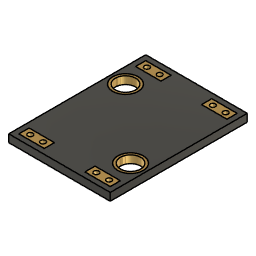
DC-DC Stepdown (Unfinished) v3 (Autodesk Fusion 360 design; units mm, degrees)
Autodesk Fusion 360 part; units mm, degrees
note: some values were not read from the file. Chosen so that the rebuilt part matches the saved one: which bodies a step acts on.
sketch "Sketch1" plane through (0, 0, 0) normal (0, 0, 1) x (1, 0, 0)
  line L0 (10, 13.5) -> (-10, 13.5)
  line L1 (-10, 13.5) -> (-10, -13.5)
  line L2 (-10, -13.5) -> (10, -13.5)
  line L3 (10, -13.5) -> (10, 13.5)
  line L4 (10, 13.5) -> (-10, -13.5) construction
  line L5 (-10, 13.5) -> (10, -13.5) construction
  line L6 (-9, -10.5) -> (-4, -10.5)
  line L7 (-4, -10.5) -> (-4, -12.5)
  line L8 (-4, -12.5) -> (-9, -12.5)
  line L9 (-9, -12.5) -> (-9, -10.5)
  line L10 (0, 13.5) -> (0, -13.5)
  line L11 (-10, 0) -> (10, 0)
  line L12 (9, -12.5) -> (4, -12.5)
  line L13 (4, -12.5) -> (4, -10.5)
  line L14 (9, -10.5) -> (9, -12.5)
  line L15 (4, -10.5) -> (9, -10.5)
  line L16 (-4, 12.5) -> (-9, 12.5)
  line L17 (-9, 12.5) -> (-9, 10.5)
  line L18 (-4, 10.5) -> (-4, 12.5)
  line L19 (-9, 10.5) -> (-4, 10.5)
  line L20 (9, 10.5) -> (4, 10.5)
  line L21 (4, 10.5) -> (4, 12.5)
  line L22 (9, 12.5) -> (9, 10.5)
  line L23 (4, 12.5) -> (9, 12.5)
  circle A0 centre (-7.75, -11.5) radius 0.5
  circle A1 centre (-5.25, -11.5) radius 0.5
  line L24 (-6.5, -10.5) -> (-6.5, -12.5)
  line L25 (6.5, -12.5) -> (6.5, -10.5)
  line L26 (6.5, 10.5) -> (6.5, 12.5)
  line L27 (-6.5, 10.5) -> (-6.5, 12.5)
  circle A2 centre (-7.75, 11.5) radius 0.5
  circle A3 centre (5.25, 11.4841) radius 0.5
  circle A4 centre (7.75, 11.4841) radius 0.5
  circle A5 centre (-5.25, 11.5) radius 0.5
  circle A6 centre (5.25, -11.4841) radius 0.5
  circle A7 centre (7.75, -11.4841) radius 0.5
  circle A8 centre (7, -6.5) radius 2
  circle A9 centre (-7, 6.5) radius 2
  circle A10 centre (-7, 6.5) radius 2.5
  circle A11 centre (7, -6.5) radius 2.5
  dimension "d1" = 20
  dimension "d2" = 27
  dimension "d3" = 1
  dimension "d4" = 5
  dimension "d5" = 1
  dimension "d6" = 2
  dimension "d9" = 1
  dimension "d10" = 1
  dimension "d11" = 1.25
  dimension "d15" = 1
  dimension "d16" = 1
  dimension "d17" = 1
  dimension "d18" = 1
  dimension "d19" = 1.25
  dimension "d20" = 1.25
  dimension "d21" = 1
  dimension "d22" = 1
  dimension "d23" = 1.25
  dimension "d31" = 1
  dimension "d32" = 1.0159
  dimension "d33" = 0.9841
  dimension "d34" = 1
  dimension "d35" = 4
  dimension "d37" = 3
  dimension "d38" = 3
  dimension "d39" = 4
  dimension "d40" = 4
  dimension "d41" = 0.5
  dimension "d42" = 0.5
  constraint horizontal L0
  constraint perpendicular L0 L1
  constraint parallel L0 L2
  constraint parallel L1 L3
  constraint coincident L4 origin
  constraint coincident L5 origin
  constraint horizontal L6
  constraint vertical L7
  constraint horizontal L8
  constraint vertical L9
  constraint midpoint L0 L10.start
  constraint midpoint L2 L10.end
  constraint midpoint L1 L11.start
  constraint midpoint L3 L11.end
  constraint horizontal L15
  constraint vertical L14
  constraint horizontal L12
  constraint vertical L13
  constraint horizontal L19
  constraint vertical L18
  constraint horizontal L16
  constraint vertical L17
  constraint horizontal L23
  constraint vertical L22
  constraint horizontal L20
  constraint vertical L21
  constraint symmetric L7 L10 L13
  constraint symmetric L6 L10 L15
  constraint symmetric L8 L10 L12
  constraint symmetric L11 L15 L20
  constraint symmetric L11 L12 L23
  constraint symmetric L6 L11 L19
  constraint symmetric L8 L11 L16
  constraint symmetric L9 L11 L17
  constraint symmetric L7 L11 L18
  constraint symmetric L11 L13 L21
  constraint midpoint L6 L24.start
  constraint midpoint L8 L24.end
  constraint symmetric A0 A1 L24
  constraint midpoint L12 L25.start
  constraint midpoint L15 L25.end
  constraint midpoint L20 L26.start
  constraint midpoint L23 L26.end
  constraint midpoint L19 L27.start
  constraint midpoint L16 L27.end
  constraint symmetric L27 A2 A5
  constraint symmetric L26 A3 A4
  constraint equal L19 L20
  constraint symmetric L25 A6 A7
  constraint equal L8 L12
  constraint equal A8 A9
  measures "d1" distance of L1.end L2.end
  measures "d2" distance of L0.end L1.end
  measures "d3" distance of L1 L9
  measures "d4" distance of L6.start L6.end
  measures "d5" distance of L2 L8
  measures "d6" distance of L6.start L8.end
  measures "d9" diameter of A0
  measures "d10" diameter of A1
  measures "d11" distance of A0.centre L24
  measures "d15" diameter of A2
  measures "d16" diameter of A3
  measures "d17" diameter of A4
  measures "d18" diameter of A5
  measures "d19" distance of L27 A2.centre
  measures "d20" distance of L26 A3.centre
  measures "d21" diameter of A6
  measures "d22" diameter of A7
  measures "d23" distance of L25 A6.centre
  measures "d31" distance of L8 A0.centre
  measures "d32" distance of L12 A6.centre
  measures "d33" distance of L20 A3.centre
  measures "d34" distance of L19 A2.centre
  measures "d35" diameter of A8
  measures "d37" distance of L1 A9.centre
  measures "d38" distance of L3 A8.centre
  measures "d39" distance of L15 A8.centre
  measures "d40" distance of L19 A9.centre
extrude "Extrude1" add sketch "Sketch1" along normal blind 1.5 contours L0 L3 L10 L11 | L0 L1 L10 L11 | L2 L3 L10 L11 | L1 L2 L10 L11 | L6 L8 L9 L24 | L6 L7 L8 L24 | L12 L14 L15 L25 | L12 L13 L15 L25 | L16 L18 L19 L27 | L16 L17 L19 L27 | L20 L22 L23 L26 | L20 L21 L23 L26 | A0 | A1 | A2 | A3 | A4 | A5 | A6 | A7 | A8 | A9 | A10 | A11 makes body 1
split "Split1" by curves path "Sketch1" along L6 L7 L8 L9 bodies 1 makes body 2 at (0, 4.5, 0)
split "Split2" by curves path "Sketch1" along L15 L14 L12 L13 bodies 2 makes body 3 at (0, 4.5, 0)
split "Split3" by curves path "Sketch1" along L23 L22 L20 L21 bodies 3 makes body 4 at (-1.3333, -3.5, 0)
split "Split4" by curves path "Sketch1" along L18 L16 L17 L19 bodies 4 makes body 5 at (-1.3333, -3.5, 0)
extrude "Extrude3" cut sketch "Sketch1" along normal blind 3 contours A0 | A1 | A2 | A3 | A4 | A5 | A6 | A7 bodies 2 3 4
extrude "Extrude4" cut sketch "Sketch1" along normal blind 4 contours A0 | A1 bodies 1
extrude "Extrude5" cut sketch "Sketch1" along normal up to surface (1.5 mm away) contours A8 | A9 bodies 5
split "Split5" by curves path "Sketch1" along A11 A10 bodies 5 makes body 6 at (-1.8252, -4.0301, 1.5) makes body 7 at (-5.0025, 6.4003, 1)
